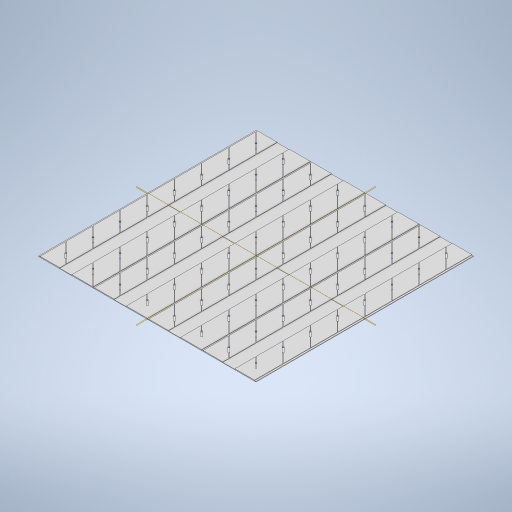
# Autodesk Inventor part: Board ReedSwitchHolder
Saved by Autodesk Inventor 2023 (Build 270158000, 158)
## iProperties
Created: 2023-04-27
Part Number: Board ReedSwitchHolder
Material: Generic
Document SubType Name: Modeling
Designer: ethan
Density: 1 g/cm^3
Appearance: Default
Author: ethan
Autodesk Inventor part; units mm, degrees
ref_plane "YZ Plane" through (0, 0, 0) normal (1, 0, 0) x (0, 1, 0)
ref_plane "XZ Plane" through (0, 0, 0) normal (0, 1, 0) x (-1, 0, 0)
ref_plane "XY Plane" through (0, 0, 0) normal (0, 0, 1) x (1, 0, 0)
sketch "Sketch1" plane through (0, 0, 0) normal (0, 1, 0) x (-1, 0, 0)
  line L0 (0, 0) -> (-649.6, 0) construction
  line L1 (-649.6, 0) -> (-649.6, -649.6) construction
  line L2 (-649.6, -649.6) -> (0, -649.6) construction
  line L3 (0, -649.6) -> (0, 0) construction
  line L4 (-45.4, -604.2) -> (-604.2, -604.2)
  line L5 (-604.2, -604.2) -> (-604.2, -45.4)
  line L6 (-604.2, -45.4) -> (-45.4, -45.4)
  line L7 (-45.4, -45.4) -> (-45.4, -604.2)
  line L8 (-96.2, -553.4) -> (-153.35, -553.4) construction
  line L9 (-153.35, -553.4) -> (-153.35, -496.25) construction
  line L10 (-153.35, -496.25) -> (-96.2, -496.25) construction
  line L11 (-96.2, -496.25) -> (-96.2, -553.4) construction
  line L12 (-96.2, -553.4) -> (-153.35, -496.25) construction
  line L13 (-118.5878, -529.2444) -> (-120.3556, -531.0122)
  line L14 (-120.3556, -531.0122) -> (-130.9622, -520.4056)
  line L15 (-130.9622, -520.4056) -> (-129.1944, -518.6378)
  line L16 (-129.1944, -518.6378) -> (-118.5878, -529.2444)
  line L17 (-118.5878, -529.2444) -> (-130.9622, -520.4056) construction
  line L18 (-120.3556, -531.0122) -> (-129.1944, -518.6378) construction
  line L19 (-177.5056, -531.0122) -> (-188.1122, -520.4056)
  line L20 (-175.7378, -529.2444) -> (-177.5056, -531.0122)
  line L21 (-186.3444, -518.6378) -> (-175.7378, -529.2444)
  line L22 (-188.1122, -520.4056) -> (-186.3444, -518.6378)
  line L23 (-234.6556, -531.0122) -> (-245.2622, -520.4056)
  line L24 (-232.8878, -529.2444) -> (-234.6556, -531.0122)
  line L25 (-243.4944, -518.6378) -> (-232.8878, -529.2444)
  line L26 (-245.2622, -520.4056) -> (-243.4944, -518.6378)
  line L27 (-291.8056, -531.0122) -> (-302.4122, -520.4056)
  line L28 (-290.0378, -529.2444) -> (-291.8056, -531.0122)
  line L29 (-300.6444, -518.6378) -> (-290.0378, -529.2444)
  line L30 (-302.4122, -520.4056) -> (-300.6444, -518.6378)
  line L31 (-348.9556, -531.0122) -> (-359.5622, -520.4056)
  line L32 (-347.1878, -529.2444) -> (-348.9556, -531.0122)
  line L33 (-357.7944, -518.6378) -> (-347.1878, -529.2444)
  line L34 (-359.5622, -520.4056) -> (-357.7944, -518.6378)
  line L35 (-406.1056, -531.0122) -> (-416.7122, -520.4056)
  line L36 (-404.3378, -529.2444) -> (-406.1056, -531.0122)
  line L37 (-414.9444, -518.6378) -> (-404.3378, -529.2444)
  line L38 (-416.7122, -520.4056) -> (-414.9444, -518.6378)
  line L39 (-463.2556, -531.0122) -> (-473.8622, -520.4056)
  line L40 (-461.4878, -529.2444) -> (-463.2556, -531.0122)
  line L41 (-472.0944, -518.6378) -> (-461.4878, -529.2444)
  line L42 (-473.8622, -520.4056) -> (-472.0944, -518.6378)
  line L43 (-520.4056, -531.0122) -> (-531.0122, -520.4056)
  line L44 (-518.6378, -529.2444) -> (-520.4056, -531.0122)
  line L45 (-529.2444, -518.6378) -> (-518.6378, -529.2444)
  line L46 (-531.0122, -520.4056) -> (-529.2444, -518.6378)
  line L47 (-120.3556, -473.8622) -> (-130.9622, -463.2556)
  line L48 (-118.5878, -472.0944) -> (-120.3556, -473.8622)
  line L49 (-129.1944, -461.4878) -> (-118.5878, -472.0944)
  line L50 (-130.9622, -463.2556) -> (-129.1944, -461.4878)
  line L51 (-177.5056, -473.8622) -> (-188.1122, -463.2556)
  line L52 (-175.7378, -472.0944) -> (-177.5056, -473.8622)
  line L53 (-186.3444, -461.4878) -> (-175.7378, -472.0944)
  line L54 (-188.1122, -463.2556) -> (-186.3444, -461.4878)
  line L55 (-234.6556, -473.8622) -> (-245.2622, -463.2556)
  line L56 (-232.8878, -472.0944) -> (-234.6556, -473.8622)
  line L57 (-243.4944, -461.4878) -> (-232.8878, -472.0944)
  line L58 (-245.2622, -463.2556) -> (-243.4944, -461.4878)
  line L59 (-291.8056, -473.8622) -> (-302.4122, -463.2556)
  line L60 (-290.0378, -472.0944) -> (-291.8056, -473.8622)
  line L61 (-300.6444, -461.4878) -> (-290.0378, -472.0944)
  line L62 (-302.4122, -463.2556) -> (-300.6444, -461.4878)
  line L63 (-348.9556, -473.8622) -> (-359.5622, -463.2556)
  line L64 (-347.1878, -472.0944) -> (-348.9556, -473.8622)
  line L65 (-357.7944, -461.4878) -> (-347.1878, -472.0944)
  line L66 (-359.5622, -463.2556) -> (-357.7944, -461.4878)
  line L67 (-406.1056, -473.8622) -> (-416.7122, -463.2556)
  line L68 (-404.3378, -472.0944) -> (-406.1056, -473.8622)
  line L69 (-414.9444, -461.4878) -> (-404.3378, -472.0944)
  line L70 (-416.7122, -463.2556) -> (-414.9444, -461.4878)
  line L71 (-463.2556, -473.8622) -> (-473.8622, -463.2556)
  line L72 (-461.4878, -472.0944) -> (-463.2556, -473.8622)
  line L73 (-472.0944, -461.4878) -> (-461.4878, -472.0944)
  line L74 (-473.8622, -463.2556) -> (-472.0944, -461.4878)
  line L75 (-520.4056, -473.8622) -> (-531.0122, -463.2556)
  line L76 (-518.6378, -472.0944) -> (-520.4056, -473.8622)
  line L77 (-529.2444, -461.4878) -> (-518.6378, -472.0944)
  line L78 (-531.0122, -463.2556) -> (-529.2444, -461.4878)
  line L79 (-120.3556, -416.7122) -> (-130.9622, -406.1056)
  line L80 (-118.5878, -414.9444) -> (-120.3556, -416.7122)
  line L81 (-129.1944, -404.3378) -> (-118.5878, -414.9444)
  line L82 (-130.9622, -406.1056) -> (-129.1944, -404.3378)
  line L83 (-177.5056, -416.7122) -> (-188.1122, -406.1056)
  line L84 (-175.7378, -414.9444) -> (-177.5056, -416.7122)
  line L85 (-186.3444, -404.3378) -> (-175.7378, -414.9444)
  line L86 (-188.1122, -406.1056) -> (-186.3444, -404.3378)
  line L87 (-234.6556, -416.7122) -> (-245.2622, -406.1056)
  line L88 (-232.8878, -414.9444) -> (-234.6556, -416.7122)
  line L89 (-243.4944, -404.3378) -> (-232.8878, -414.9444)
  line L90 (-245.2622, -406.1056) -> (-243.4944, -404.3378)
  line L91 (-291.8056, -416.7122) -> (-302.4122, -406.1056)
  line L92 (-290.0378, -414.9444) -> (-291.8056, -416.7122)
  line L93 (-300.6444, -404.3378) -> (-290.0378, -414.9444)
  line L94 (-302.4122, -406.1056) -> (-300.6444, -404.3378)
  line L95 (-348.9556, -416.7122) -> (-359.5622, -406.1056)
  line L96 (-347.1878, -414.9444) -> (-348.9556, -416.7122)
  line L97 (-357.7944, -404.3378) -> (-347.1878, -414.9444)
  line L98 (-359.5622, -406.1056) -> (-357.7944, -404.3378)
  line L99 (-406.1056, -416.7122) -> (-416.7122, -406.1056)
  line L100 (-404.3378, -414.9444) -> (-406.1056, -416.7122)
  line L101 (-414.9444, -404.3378) -> (-404.3378, -414.9444)
  line L102 (-416.7122, -406.1056) -> (-414.9444, -404.3378)
  line L103 (-463.2556, -416.7122) -> (-473.8622, -406.1056)
  line L104 (-461.4878, -414.9444) -> (-463.2556, -416.7122)
  line L105 (-472.0944, -404.3378) -> (-461.4878, -414.9444)
  line L106 (-473.8622, -406.1056) -> (-472.0944, -404.3378)
  line L107 (-520.4056, -416.7122) -> (-531.0122, -406.1056)
  line L108 (-518.6378, -414.9444) -> (-520.4056, -416.7122)
  line L109 (-529.2444, -404.3378) -> (-518.6378, -414.9444)
  line L110 (-531.0122, -406.1056) -> (-529.2444, -404.3378)
  line L111 (-120.3556, -359.5622) -> (-130.9622, -348.9556)
  line L112 (-118.5878, -357.7944) -> (-120.3556, -359.5622)
  line L113 (-129.1944, -347.1878) -> (-118.5878, -357.7944)
  line L114 (-130.9622, -348.9556) -> (-129.1944, -347.1878)
  line L115 (-177.5056, -359.5622) -> (-188.1122, -348.9556)
  line L116 (-175.7378, -357.7944) -> (-177.5056, -359.5622)
  line L117 (-186.3444, -347.1878) -> (-175.7378, -357.7944)
  line L118 (-188.1122, -348.9556) -> (-186.3444, -347.1878)
  line L119 (-234.6556, -359.5622) -> (-245.2622, -348.9556)
  line L120 (-232.8878, -357.7944) -> (-234.6556, -359.5622)
  line L121 (-243.4944, -347.1878) -> (-232.8878, -357.7944)
  line L122 (-245.2622, -348.9556) -> (-243.4944, -347.1878)
  line L123 (-291.8056, -359.5622) -> (-302.4122, -348.9556)
  line L124 (-290.0378, -357.7944) -> (-291.8056, -359.5622)
  line L125 (-300.6444, -347.1878) -> (-290.0378, -357.7944)
  line L126 (-302.4122, -348.9556) -> (-300.6444, -347.1878)
  line L127 (-348.9556, -359.5622) -> (-359.5622, -348.9556)
  line L128 (-347.1878, -357.7944) -> (-348.9556, -359.5622)
  line L129 (-357.7944, -347.1878) -> (-347.1878, -357.7944)
  line L130 (-359.5622, -348.9556) -> (-357.7944, -347.1878)
  line L131 (-406.1056, -359.5622) -> (-416.7122, -348.9556)
  line L132 (-404.3378, -357.7944) -> (-406.1056, -359.5622)
  line L133 (-414.9444, -347.1878) -> (-404.3378, -357.7944)
  line L134 (-416.7122, -348.9556) -> (-414.9444, -347.1878)
  line L135 (-463.2556, -359.5622) -> (-473.8622, -348.9556)
  line L136 (-461.4878, -357.7944) -> (-463.2556, -359.5622)
  line L137 (-472.0944, -347.1878) -> (-461.4878, -357.7944)
  line L138 (-473.8622, -348.9556) -> (-472.0944, -347.1878)
  line L139 (-520.4056, -359.5622) -> (-531.0122, -348.9556)
  line L140 (-518.6378, -357.7944) -> (-520.4056, -359.5622)
  line L141 (-529.2444, -347.1878) -> (-518.6378, -357.7944)
  line L142 (-531.0122, -348.9556) -> (-529.2444, -347.1878)
  line L143 (-120.3556, -302.4122) -> (-130.9622, -291.8056)
  line L144 (-118.5878, -300.6444) -> (-120.3556, -302.4122)
  line L145 (-129.1944, -290.0378) -> (-118.5878, -300.6444)
  line L146 (-130.9622, -291.8056) -> (-129.1944, -290.0378)
  line L147 (-177.5056, -302.4122) -> (-188.1122, -291.8056)
  line L148 (-175.7378, -300.6444) -> (-177.5056, -302.4122)
  line L149 (-186.3444, -290.0378) -> (-175.7378, -300.6444)
  line L150 (-188.1122, -291.8056) -> (-186.3444, -290.0378)
  line L151 (-234.6556, -302.4122) -> (-245.2622, -291.8056)
  line L152 (-232.8878, -300.6444) -> (-234.6556, -302.4122)
  line L153 (-243.4944, -290.0378) -> (-232.8878, -300.6444)
  line L154 (-245.2622, -291.8056) -> (-243.4944, -290.0378)
  line L155 (-291.8056, -302.4122) -> (-302.4122, -291.8056)
  line L156 (-290.0378, -300.6444) -> (-291.8056, -302.4122)
  line L157 (-300.6444, -290.0378) -> (-290.0378, -300.6444)
  line L158 (-302.4122, -291.8056) -> (-300.6444, -290.0378)
  line L159 (-348.9556, -302.4122) -> (-359.5622, -291.8056)
  line L160 (-347.1878, -300.6444) -> (-348.9556, -302.4122)
  line L161 (-357.7944, -290.0378) -> (-347.1878, -300.6444)
  line L162 (-359.5622, -291.8056) -> (-357.7944, -290.0378)
  line L163 (-406.1056, -302.4122) -> (-416.7122, -291.8056)
  line L164 (-404.3378, -300.6444) -> (-406.1056, -302.4122)
  line L165 (-414.9444, -290.0378) -> (-404.3378, -300.6444)
  line L166 (-416.7122, -291.8056) -> (-414.9444, -290.0378)
  line L167 (-463.2556, -302.4122) -> (-473.8622, -291.8056)
  line L168 (-461.4878, -300.6444) -> (-463.2556, -302.4122)
  line L169 (-472.0944, -290.0378) -> (-461.4878, -300.6444)
  line L170 (-473.8622, -291.8056) -> (-472.0944, -290.0378)
  line L171 (-520.4056, -302.4122) -> (-531.0122, -291.8056)
  line L172 (-518.6378, -300.6444) -> (-520.4056, -302.4122)
  line L173 (-529.2444, -290.0378) -> (-518.6378, -300.6444)
  line L174 (-531.0122, -291.8056) -> (-529.2444, -290.0378)
  line L175 (-120.3556, -245.2622) -> (-130.9622, -234.6556)
  line L176 (-118.5878, -243.4944) -> (-120.3556, -245.2622)
  line L177 (-129.1944, -232.8878) -> (-118.5878, -243.4944)
  line L178 (-130.9622, -234.6556) -> (-129.1944, -232.8878)
  line L179 (-177.5056, -245.2622) -> (-188.1122, -234.6556)
  line L180 (-175.7378, -243.4944) -> (-177.5056, -245.2622)
  line L181 (-186.3444, -232.8878) -> (-175.7378, -243.4944)
  line L182 (-188.1122, -234.6556) -> (-186.3444, -232.8878)
  line L183 (-234.6556, -245.2622) -> (-245.2622, -234.6556)
  line L184 (-232.8878, -243.4944) -> (-234.6556, -245.2622)
  line L185 (-243.4944, -232.8878) -> (-232.8878, -243.4944)
  line L186 (-245.2622, -234.6556) -> (-243.4944, -232.8878)
  line L187 (-291.8056, -245.2622) -> (-302.4122, -234.6556)
  line L188 (-290.0378, -243.4944) -> (-291.8056, -245.2622)
  line L189 (-300.6444, -232.8878) -> (-290.0378, -243.4944)
  line L190 (-302.4122, -234.6556) -> (-300.6444, -232.8878)
  line L191 (-348.9556, -245.2622) -> (-359.5622, -234.6556)
  line L192 (-347.1878, -243.4944) -> (-348.9556, -245.2622)
  line L193 (-357.7944, -232.8878) -> (-347.1878, -243.4944)
  line L194 (-359.5622, -234.6556) -> (-357.7944, -232.8878)
  line L195 (-406.1056, -245.2622) -> (-416.7122, -234.6556)
  line L196 (-404.3378, -243.4944) -> (-406.1056, -245.2622)
  line L197 (-414.9444, -232.8878) -> (-404.3378, -243.4944)
  line L198 (-416.7122, -234.6556) -> (-414.9444, -232.8878)
  line L199 (-463.2556, -245.2622) -> (-473.8622, -234.6556)
  line L200 (-461.4878, -243.4944) -> (-463.2556, -245.2622)
  line L201 (-472.0944, -232.8878) -> (-461.4878, -243.4944)
  line L202 (-473.8622, -234.6556) -> (-472.0944, -232.8878)
  line L203 (-520.4056, -245.2622) -> (-531.0122, -234.6556)
  line L204 (-518.6378, -243.4944) -> (-520.4056, -245.2622)
  line L205 (-529.2444, -232.8878) -> (-518.6378, -243.4944)
  line L206 (-531.0122, -234.6556) -> (-529.2444, -232.8878)
  line L207 (-120.3556, -188.1122) -> (-130.9622, -177.5056)
  line L208 (-118.5878, -186.3444) -> (-120.3556, -188.1122)
  line L209 (-129.1944, -175.7378) -> (-118.5878, -186.3444)
  line L210 (-130.9622, -177.5056) -> (-129.1944, -175.7378)
  line L211 (-177.5056, -188.1122) -> (-188.1122, -177.5056)
  line L212 (-175.7378, -186.3444) -> (-177.5056, -188.1122)
  line L213 (-186.3444, -175.7378) -> (-175.7378, -186.3444)
  line L214 (-188.1122, -177.5056) -> (-186.3444, -175.7378)
  line L215 (-234.6556, -188.1122) -> (-245.2622, -177.5056)
  line L216 (-232.8878, -186.3444) -> (-234.6556, -188.1122)
  line L217 (-243.4944, -175.7378) -> (-232.8878, -186.3444)
  line L218 (-245.2622, -177.5056) -> (-243.4944, -175.7378)
  line L219 (-291.8056, -188.1122) -> (-302.4122, -177.5056)
  line L220 (-290.0378, -186.3444) -> (-291.8056, -188.1122)
  line L221 (-300.6444, -175.7378) -> (-290.0378, -186.3444)
  line L222 (-302.4122, -177.5056) -> (-300.6444, -175.7378)
  line L223 (-348.9556, -188.1122) -> (-359.5622, -177.5056)
  line L224 (-347.1878, -186.3444) -> (-348.9556, -188.1122)
  line L225 (-357.7944, -175.7378) -> (-347.1878, -186.3444)
  line L226 (-359.5622, -177.5056) -> (-357.7944, -175.7378)
  line L227 (-406.1056, -188.1122) -> (-416.7122, -177.5056)
  line L228 (-404.3378, -186.3444) -> (-406.1056, -188.1122)
  line L229 (-414.9444, -175.7378) -> (-404.3378, -186.3444)
  line L230 (-416.7122, -177.5056) -> (-414.9444, -175.7378)
  line L231 (-463.2556, -188.1122) -> (-473.8622, -177.5056)
  line L232 (-461.4878, -186.3444) -> (-463.2556, -188.1122)
  line L233 (-472.0944, -175.7378) -> (-461.4878, -186.3444)
  line L234 (-473.8622, -177.5056) -> (-472.0944, -175.7378)
  line L235 (-520.4056, -188.1122) -> (-531.0122, -177.5056)
  line L236 (-518.6378, -186.3444) -> (-520.4056, -188.1122)
  line L237 (-529.2444, -175.7378) -> (-518.6378, -186.3444)
  line L238 (-531.0122, -177.5056) -> (-529.2444, -175.7378)
  line L239 (-120.3556, -130.9622) -> (-130.9622, -120.3556)
  line L240 (-118.5878, -129.1944) -> (-120.3556, -130.9622)
  line L241 (-129.1944, -118.5878) -> (-118.5878, -129.1944)
  line L242 (-130.9622, -120.3556) -> (-129.1944, -118.5878)
  line L243 (-177.5056, -130.9622) -> (-188.1122, -120.3556)
  line L244 (-175.7378, -129.1944) -> (-177.5056, -130.9622)
  line L245 (-186.3444, -118.5878) -> (-175.7378, -129.1944)
  line L246 (-188.1122, -120.3556) -> (-186.3444, -118.5878)
  line L247 (-234.6556, -130.9622) -> (-245.2622, -120.3556)
  line L248 (-232.8878, -129.1944) -> (-234.6556, -130.9622)
  line L249 (-243.4944, -118.5878) -> (-232.8878, -129.1944)
  line L250 (-245.2622, -120.3556) -> (-243.4944, -118.5878)
  line L251 (-291.8056, -130.9622) -> (-302.4122, -120.3556)
  line L252 (-290.0378, -129.1944) -> (-291.8056, -130.9622)
  line L253 (-300.6444, -118.5878) -> (-290.0378, -129.1944)
  line L254 (-302.4122, -120.3556) -> (-300.6444, -118.5878)
  line L255 (-348.9556, -130.9622) -> (-359.5622, -120.3556)
  line L256 (-347.1878, -129.1944) -> (-348.9556, -130.9622)
  line L257 (-357.7944, -118.5878) -> (-347.1878, -129.1944)
  line L258 (-359.5622, -120.3556) -> (-357.7944, -118.5878)
  line L259 (-406.1056, -130.9622) -> (-416.7122, -120.3556)
  line L260 (-404.3378, -129.1944) -> (-406.1056, -130.9622)
  line L261 (-414.9444, -118.5878) -> (-404.3378, -129.1944)
  line L262 (-416.7122, -120.3556) -> (-414.9444, -118.5878)
  line L263 (-463.2556, -130.9622) -> (-473.8622, -120.3556)
  line L264 (-461.4878, -129.1944) -> (-463.2556, -130.9622)
  line L265 (-472.0944, -118.5878) -> (-461.4878, -129.1944)
  line L266 (-473.8622, -120.3556) -> (-472.0944, -118.5878)
  line L267 (-520.4056, -130.9622) -> (-531.0122, -120.3556)
  line L268 (-518.6378, -129.1944) -> (-520.4056, -130.9622)
  line L269 (-529.2444, -118.5878) -> (-518.6378, -129.1944)
  line L270 (-531.0122, -120.3556) -> (-529.2444, -118.5878)
  line L271 (-96.2, -553.4) -> (-553.4, -553.4)
  line L272 (-553.4, -553.4) -> (-553.4, -96.2)
  line L273 (-553.4, -96.2) -> (-96.2, -96.2)
  line L274 (-96.2, -96.2) -> (-96.2, -553.4)
  line L275 (-553.4, -324.8) -> (-96.2, -324.8)
  line L276 (-324.8, -553.4) -> (-324.8, -96.2)
  point P0 (-124.775, -524.825)
  dimension "d0" = 649.6
  dimension "d1" = 649.6
  dimension "d10" = 45.4
  dimension "d11" = 50.8
  dimension "d12" = 50.8
  dimension "d15" = 57.15
  dimension "d16" = 57.15
  dimension "d17" = 2.5
  dimension "d18" = 15
  dimension "d22" = 57.15
  dimension "d25" = 57.15
  dimension "d30" = 50.8
  constraints: 554 end point, 10 parallel, 7 midpoint, 6 perpendicular, 3 horizontal, 1 vertical, 510 other
  measures "d0" distance of L2.end L1.end
  measures "d1" distance of L1.end L0.end
  measures "d10" distance between parallel lines of L2 L4
  measures "d11" distance from line of L4 L8.start
  measures "d12" distance from line of L7 L8.start
  measures "d15" distance of L9.end L10.end
  measures "d16" distance of L8.end L9.end
  measures "d17" distance of L13.start L13.end
  measures "d18" distance of L13.end L14.end
  measures "d22" distance of L13.end L19.start
  measures "d25" distance of L13.end L47.start
  measures "d30" distance between parallel lines of L7 L274
extrude "Extrusion1" add sketch "Sketch1" along normal blind 2 contours L271 L276 L275 L274 | L271 L272 L275 L276 | L275 L276 L273 L274 | L275 L272 L273 L276
sketch "Sketch2" plane through (0, 2, 0) normal (0, 1, 0) x (1, 0, 0)
  line L0 (553.4, 553.4) -> (96.2, 553.4) projected
  line L1 (96.2, 553.4) -> (99.375, 553.4)
  line L2 (99.375, 553.4) -> (99.375, 96.2)
  line L3 (99.375, 96.2) -> (96.2, 96.2)
  line L4 (96.2, 96.2) -> (96.2, 553.4)
  line L5 (553.4, 96.2) -> (553.4, 553.4) projected
  line L6 (140.65, 553.4) -> (166.05, 553.4)
  line L7 (166.05, 553.4) -> (166.05, 96.2)
  line L8 (166.05, 96.2) -> (140.65, 96.2)
  line L9 (140.65, 96.2) -> (140.65, 553.4)
  line L10 (280.35, 553.4) -> (280.35, 96.2)
  line L11 (254.95, 96.2) -> (254.95, 553.4)
  line L12 (254.95, 553.4) -> (280.35, 553.4)
  line L13 (213.675, 553.4) -> (213.675, 96.2)
  line L14 (210.5, 96.2) -> (210.5, 553.4)
  line L15 (210.5, 553.4) -> (213.675, 553.4)
  line L16 (280.35, 96.2) -> (254.95, 96.2)
  line L17 (213.675, 96.2) -> (210.5, 96.2)
  line L18 (394.65, 553.4) -> (394.65, 96.2)
  line L19 (369.25, 96.2) -> (369.25, 553.4)
  line L20 (369.25, 553.4) -> (394.65, 553.4)
  line L21 (327.975, 553.4) -> (327.975, 96.2)
  line L22 (324.8, 96.2) -> (324.8, 553.4)
  line L23 (324.8, 553.4) -> (327.975, 553.4)
  line L24 (394.65, 96.2) -> (369.25, 96.2)
  line L25 (327.975, 96.2) -> (324.8, 96.2)
  line L26 (508.95, 553.4) -> (508.95, 96.2)
  line L27 (483.55, 96.2) -> (483.55, 553.4)
  line L28 (483.55, 553.4) -> (508.95, 553.4)
  line L29 (442.275, 553.4) -> (442.275, 96.2)
  line L30 (439.1, 96.2) -> (439.1, 553.4)
  line L31 (439.1, 553.4) -> (442.275, 553.4)
  line L32 (508.95, 96.2) -> (483.55, 96.2)
  line L33 (442.275, 96.2) -> (439.1, 96.2)
  line L34 (553.4, 553.4) -> (550.225, 553.4)
  line L35 (550.225, 553.4) -> (550.225, 96.2)
  line L36 (550.225, 96.2) -> (553.4, 96.2)
  line L37 (553.4, 96.2) -> (553.4, 553.4)
  line L38 (118.5878, 529.2444) -> (120.3556, 531.0122) construction
  line L39 (119.4717, 530.1283) -> (99.375, 550.225) construction
  line L40 (130.9622, 520.4056) -> (129.1944, 518.6378) construction
  line L41 (130.0783, 519.5217) -> (140.65, 508.95) construction
  line L42 (119.8253, 530.4819) -> (99.375, 550.9321)
  line L43 (119.1181, 529.7747) -> (99.375, 549.5179)
  line L44 (130.4319, 519.8753) -> (140.65, 509.6571)
  line L45 (129.7247, 519.1681) -> (140.65, 508.2429)
  line L46 (118.5878, 529.2444) -> (120.3556, 531.0122) construction
  line L47 (130.9622, 520.4056) -> (129.1944, 518.6378) construction
  line L48 (234.1253, 530.4819) -> (213.675, 550.9321)
  line L49 (233.4181, 529.7747) -> (213.675, 549.5179)
  line L50 (244.7319, 519.8753) -> (254.95, 509.6571)
  line L51 (244.0247, 519.1681) -> (254.95, 508.2429)
  line L52 (348.4253, 530.4819) -> (327.975, 550.9321)
  line L53 (347.7181, 529.7747) -> (327.975, 549.5179)
  line L54 (359.0319, 519.8753) -> (369.25, 509.6571)
  line L55 (358.3247, 519.1681) -> (369.25, 508.2429)
  line L56 (462.7253, 530.4819) -> (442.275, 550.9321)
  line L57 (462.0181, 529.7747) -> (442.275, 549.5179)
  line L58 (473.3319, 519.8753) -> (483.55, 509.6571)
  line L59 (472.6247, 519.1681) -> (483.55, 508.2429)
  line L60 (119.8253, 473.3319) -> (99.375, 493.7821)
  line L61 (119.1181, 472.6247) -> (99.375, 492.3679)
  line L62 (130.4319, 462.7253) -> (140.65, 452.5071)
  line L63 (129.7247, 462.0181) -> (140.65, 451.0929)
  line L64 (234.1253, 473.3319) -> (213.675, 493.7821)
  line L65 (233.4181, 472.6247) -> (213.675, 492.3679)
  line L66 (244.7319, 462.7253) -> (254.95, 452.5071)
  line L67 (244.0247, 462.0181) -> (254.95, 451.0929)
  line L68 (348.4253, 473.3319) -> (327.975, 493.7821)
  line L69 (347.7181, 472.6247) -> (327.975, 492.3679)
  line L70 (359.0319, 462.7253) -> (369.25, 452.5071)
  line L71 (358.3247, 462.0181) -> (369.25, 451.0929)
  line L72 (462.7253, 473.3319) -> (442.275, 493.7821)
  line L73 (462.0181, 472.6247) -> (442.275, 492.3679)
  line L74 (473.3319, 462.7253) -> (483.55, 452.5071)
  line L75 (472.6247, 462.0181) -> (483.55, 451.0929)
  line L76 (119.8253, 416.1819) -> (99.375, 436.6321)
  line L77 (119.1181, 415.4747) -> (99.375, 435.2179)
  line L78 (130.4319, 405.5753) -> (140.65, 395.3571)
  line L79 (129.7247, 404.8681) -> (140.65, 393.9429)
  line L80 (234.1253, 416.1819) -> (213.675, 436.6321)
  line L81 (233.4181, 415.4747) -> (213.675, 435.2179)
  line L82 (244.7319, 405.5753) -> (254.95, 395.3571)
  line L83 (244.0247, 404.8681) -> (254.95, 393.9429)
  line L84 (348.4253, 416.1819) -> (327.975, 436.6321)
  line L85 (347.7181, 415.4747) -> (327.975, 435.2179)
  line L86 (359.0319, 405.5753) -> (369.25, 395.3571)
  line L87 (358.3247, 404.8681) -> (369.25, 393.9429)
  line L88 (462.7253, 416.1819) -> (442.275, 436.6321)
  line L89 (462.0181, 415.4747) -> (442.275, 435.2179)
  line L90 (473.3319, 405.5753) -> (483.55, 395.3571)
  line L91 (472.6247, 404.8681) -> (483.55, 393.9429)
  line L92 (119.8253, 359.0319) -> (99.375, 379.4821)
  line L93 (119.1181, 358.3247) -> (99.375, 378.0679)
  line L94 (130.4319, 348.4253) -> (140.65, 338.2071)
  line L95 (129.7247, 347.7181) -> (140.65, 336.7929)
  line L96 (234.1253, 359.0319) -> (213.675, 379.4821)
  line L97 (233.4181, 358.3247) -> (213.675, 378.0679)
  line L98 (244.7319, 348.4253) -> (254.95, 338.2071)
  line L99 (244.0247, 347.7181) -> (254.95, 336.7929)
  line L100 (348.4253, 359.0319) -> (327.975, 379.4821)
  line L101 (347.7181, 358.3247) -> (327.975, 378.0679)
  line L102 (359.0319, 348.4253) -> (369.25, 338.2071)
  line L103 (358.3247, 347.7181) -> (369.25, 336.7929)
  line L104 (462.7253, 359.0319) -> (442.275, 379.4821)
  line L105 (462.0181, 358.3247) -> (442.275, 378.0679)
  line L106 (473.3319, 348.4253) -> (483.55, 338.2071)
  line L107 (472.6247, 347.7181) -> (483.55, 336.7929)
  line L108 (119.8253, 301.8819) -> (99.375, 322.3321)
  line L109 (119.1181, 301.1747) -> (99.375, 320.9179)
  line L110 (130.4319, 291.2753) -> (140.65, 281.0571)
  line L111 (129.7247, 290.5681) -> (140.65, 279.6429)
  line L112 (234.1253, 301.8819) -> (213.675, 322.3321)
  line L113 (233.4181, 301.1747) -> (213.675, 320.9179)
  line L114 (244.7319, 291.2753) -> (254.95, 281.0571)
  line L115 (244.0247, 290.5681) -> (254.95, 279.6429)
  line L116 (348.4253, 301.8819) -> (327.975, 322.3321)
  line L117 (347.7181, 301.1747) -> (327.975, 320.9179)
  line L118 (359.0319, 291.2753) -> (369.25, 281.0571)
  line L119 (358.3247, 290.5681) -> (369.25, 279.6429)
  line L120 (462.7253, 301.8819) -> (442.275, 322.3321)
  line L121 (462.0181, 301.1747) -> (442.275, 320.9179)
  line L122 (473.3319, 291.2753) -> (483.55, 281.0571)
  line L123 (472.6247, 290.5681) -> (483.55, 279.6429)
  line L124 (119.8253, 244.7319) -> (99.375, 265.1821)
  line L125 (119.1181, 244.0247) -> (99.375, 263.7679)
  line L126 (130.4319, 234.1253) -> (140.65, 223.9071)
  line L127 (129.7247, 233.4181) -> (140.65, 222.4929)
  line L128 (234.1253, 244.7319) -> (213.675, 265.1821)
  line L129 (233.4181, 244.0247) -> (213.675, 263.7679)
  line L130 (244.7319, 234.1253) -> (254.95, 223.9071)
  line L131 (244.0247, 233.4181) -> (254.95, 222.4929)
  line L132 (348.4253, 244.7319) -> (327.975, 265.1821)
  line L133 (347.7181, 244.0247) -> (327.975, 263.7679)
  line L134 (359.0319, 234.1253) -> (369.25, 223.9071)
  line L135 (358.3247, 233.4181) -> (369.25, 222.4929)
  line L136 (462.7253, 244.7319) -> (442.275, 265.1821)
  line L137 (462.0181, 244.0247) -> (442.275, 263.7679)
  line L138 (473.3319, 234.1253) -> (483.55, 223.9071)
  line L139 (472.6247, 233.4181) -> (483.55, 222.4929)
  line L140 (119.8253, 187.5819) -> (99.375, 208.0321)
  line L141 (119.1181, 186.8747) -> (99.375, 206.6179)
  line L142 (130.4319, 176.9753) -> (140.65, 166.7571)
  line L143 (129.7247, 176.2681) -> (140.65, 165.3429)
  line L144 (234.1253, 187.5819) -> (213.675, 208.0321)
  line L145 (233.4181, 186.8747) -> (213.675, 206.6179)
  line L146 (244.7319, 176.9753) -> (254.95, 166.7571)
  line L147 (244.0247, 176.2681) -> (254.95, 165.3429)
  line L148 (348.4253, 187.5819) -> (327.975, 208.0321)
  line L149 (347.7181, 186.8747) -> (327.975, 206.6179)
  line L150 (359.0319, 176.9753) -> (369.25, 166.7571)
  line L151 (358.3247, 176.2681) -> (369.25, 165.3429)
  line L152 (462.7253, 187.5819) -> (442.275, 208.0321)
  line L153 (462.0181, 186.8747) -> (442.275, 206.6179)
  line L154 (473.3319, 176.9753) -> (483.55, 166.7571)
  line L155 (472.6247, 176.2681) -> (483.55, 165.3429)
  line L156 (119.8253, 130.4319) -> (99.375, 150.8821)
  line L157 (119.1181, 129.7247) -> (99.375, 149.4679)
  line L158 (130.4319, 119.8253) -> (140.65, 109.6071)
  line L159 (129.7247, 119.1181) -> (140.65, 108.1929)
  line L160 (234.1253, 130.4319) -> (213.675, 150.8821)
  line L161 (233.4181, 129.7247) -> (213.675, 149.4679)
  line L162 (244.7319, 119.8253) -> (254.95, 109.6071)
  line L163 (244.0247, 119.1181) -> (254.95, 108.1929)
  line L164 (348.4253, 130.4319) -> (327.975, 150.8821)
  line L165 (347.7181, 129.7247) -> (327.975, 149.4679)
  line L166 (359.0319, 119.8253) -> (369.25, 109.6071)
  line L167 (358.3247, 119.1181) -> (369.25, 108.1929)
  line L168 (462.7253, 130.4319) -> (442.275, 150.8821)
  line L169 (462.0181, 129.7247) -> (442.275, 149.4679)
  line L170 (473.3319, 119.8253) -> (483.55, 109.6071)
  line L171 (472.6247, 119.1181) -> (483.55, 108.1929)
  line L172 (175.7378, 529.2444) -> (177.5056, 531.0122) construction
  line L173 (176.6217, 530.1283) -> (166.05, 540.7) construction
  line L174 (188.1122, 520.4056) -> (186.3444, 518.6378) construction
  line L175 (187.2283, 519.5217) -> (210.5, 496.25) construction
  line L176 (176.9753, 530.4819) -> (166.05, 541.4071)
  line L177 (176.2681, 529.7747) -> (166.05, 539.9929)
  line L178 (187.5819, 519.8753) -> (210.5, 496.9571)
  line L179 (186.8747, 519.1681) -> (210.5, 495.5429)
  line L180 (291.2753, 530.4819) -> (280.35, 541.4071)
  line L181 (290.5681, 529.7747) -> (280.35, 539.9929)
  line L182 (301.8819, 519.8753) -> (324.8, 496.9571)
  line L183 (301.1747, 519.1681) -> (324.8, 495.5429)
  line L184 (405.5753, 530.4819) -> (394.65, 541.4071)
  line L185 (404.8681, 529.7747) -> (394.65, 539.9929)
  line L186 (416.1819, 519.8753) -> (439.1, 496.9571)
  line L187 (415.4747, 519.1681) -> (439.1, 495.5429)
  line L188 (519.8753, 530.4819) -> (508.95, 541.4071)
  line L189 (519.1681, 529.7747) -> (508.95, 539.9929)
  line L190 (530.4819, 519.8753) -> (553.4, 496.9571)
  line L191 (529.7747, 519.1681) -> (553.4, 495.5429)
  line L192 (176.9753, 473.3319) -> (166.05, 484.2571)
  line L193 (176.2681, 472.6247) -> (166.05, 482.8429)
  line L194 (187.5819, 462.7253) -> (210.5, 439.8071)
  line L195 (186.8747, 462.0181) -> (210.5, 438.3929)
  line L196 (291.2753, 473.3319) -> (280.35, 484.2571)
  line L197 (290.5681, 472.6247) -> (280.35, 482.8429)
  line L198 (301.8819, 462.7253) -> (324.8, 439.8071)
  line L199 (301.1747, 462.0181) -> (324.8, 438.3929)
  line L200 (405.5753, 473.3319) -> (394.65, 484.2571)
  line L201 (404.8681, 472.6247) -> (394.65, 482.8429)
  line L202 (416.1819, 462.7253) -> (439.1, 439.8071)
  line L203 (415.4747, 462.0181) -> (439.1, 438.3929)
  line L204 (519.8753, 473.3319) -> (508.95, 484.2571)
  line L205 (519.1681, 472.6247) -> (508.95, 482.8429)
  line L206 (530.4819, 462.7253) -> (553.4, 439.8071)
  line L207 (529.7747, 462.0181) -> (553.4, 438.3929)
  line L208 (176.9753, 416.1819) -> (166.05, 427.1071)
  line L209 (176.2681, 415.4747) -> (166.05, 425.6929)
  line L210 (187.5819, 405.5753) -> (210.5, 382.6571)
  line L211 (186.8747, 404.8681) -> (210.5, 381.2429)
  line L212 (291.2753, 416.1819) -> (280.35, 427.1071)
  line L213 (290.5681, 415.4747) -> (280.35, 425.6929)
  line L214 (301.8819, 405.5753) -> (324.8, 382.6571)
  line L215 (301.1747, 404.8681) -> (324.8, 381.2429)
  line L216 (405.5753, 416.1819) -> (394.65, 427.1071)
  line L217 (404.8681, 415.4747) -> (394.65, 425.6929)
  line L218 (416.1819, 405.5753) -> (439.1, 382.6571)
  line L219 (415.4747, 404.8681) -> (439.1, 381.2429)
  line L220 (519.8753, 416.1819) -> (508.95, 427.1071)
  line L221 (519.1681, 415.4747) -> (508.95, 425.6929)
  line L222 (530.4819, 405.5753) -> (553.4, 382.6571)
  line L223 (529.7747, 404.8681) -> (553.4, 381.2429)
  line L224 (176.9753, 359.0319) -> (166.05, 369.9571)
  line L225 (176.2681, 358.3247) -> (166.05, 368.5429)
  line L226 (187.5819, 348.4253) -> (210.5, 325.5071)
  line L227 (186.8747, 347.7181) -> (210.5, 324.0929)
  line L228 (291.2753, 359.0319) -> (280.35, 369.9571)
  line L229 (290.5681, 358.3247) -> (280.35, 368.5429)
  line L230 (301.8819, 348.4253) -> (324.8, 325.5071)
  line L231 (301.1747, 347.7181) -> (324.8, 324.0929)
  line L232 (405.5753, 359.0319) -> (394.65, 369.9571)
  line L233 (404.8681, 358.3247) -> (394.65, 368.5429)
  line L234 (416.1819, 348.4253) -> (439.1, 325.5071)
  line L235 (415.4747, 347.7181) -> (439.1, 324.0929)
  line L236 (519.8753, 359.0319) -> (508.95, 369.9571)
  line L237 (519.1681, 358.3247) -> (508.95, 368.5429)
  line L238 (530.4819, 348.4253) -> (553.4, 325.5071)
  line L239 (529.7747, 347.7181) -> (553.4, 324.0929)
  line L240 (176.9753, 301.8819) -> (166.05, 312.8071)
  line L241 (176.2681, 301.1747) -> (166.05, 311.3929)
  line L242 (187.5819, 291.2753) -> (210.5, 268.3571)
  line L243 (186.8747, 290.5681) -> (210.5, 266.9429)
  line L244 (291.2753, 301.8819) -> (280.35, 312.8071)
  line L245 (290.5681, 301.1747) -> (280.35, 311.3929)
  line L246 (301.8819, 291.2753) -> (324.8, 268.3571)
  line L247 (301.1747, 290.5681) -> (324.8, 266.9429)
  line L248 (405.5753, 301.8819) -> (394.65, 312.8071)
  line L249 (404.8681, 301.1747) -> (394.65, 311.3929)
  line L250 (416.1819, 291.2753) -> (439.1, 268.3571)
  line L251 (415.4747, 290.5681) -> (439.1, 266.9429)
  line L252 (519.8753, 301.8819) -> (508.95, 312.8071)
  line L253 (519.1681, 301.1747) -> (508.95, 311.3929)
  line L254 (530.4819, 291.2753) -> (553.4, 268.3571)
  line L255 (529.7747, 290.5681) -> (553.4, 266.9429)
  line L256 (176.9753, 244.7319) -> (166.05, 255.6571)
  line L257 (176.2681, 244.0247) -> (166.05, 254.2429)
  line L258 (187.5819, 234.1253) -> (210.5, 211.2071)
  line L259 (186.8747, 233.4181) -> (210.5, 209.7929)
  line L260 (291.2753, 244.7319) -> (280.35, 255.6571)
  line L261 (290.5681, 244.0247) -> (280.35, 254.2429)
  line L262 (301.8819, 234.1253) -> (324.8, 211.2071)
  line L263 (301.1747, 233.4181) -> (324.8, 209.7929)
  line L264 (405.5753, 244.7319) -> (394.65, 255.6571)
  line L265 (404.8681, 244.0247) -> (394.65, 254.2429)
  line L266 (416.1819, 234.1253) -> (439.1, 211.2071)
  line L267 (415.4747, 233.4181) -> (439.1, 209.7929)
  line L268 (519.8753, 244.7319) -> (508.95, 255.6571)
  line L269 (519.1681, 244.0247) -> (508.95, 254.2429)
  line L270 (530.4819, 234.1253) -> (553.4, 211.2071)
  line L271 (529.7747, 233.4181) -> (553.4, 209.7929)
  line L272 (176.9753, 187.5819) -> (166.05, 198.5071)
  line L273 (176.2681, 186.8747) -> (166.05, 197.0929)
  line L274 (187.5819, 176.9753) -> (210.5, 154.0571)
  line L275 (186.8747, 176.2681) -> (210.5, 152.6429)
  line L276 (291.2753, 187.5819) -> (280.35, 198.5071)
  line L277 (290.5681, 186.8747) -> (280.35, 197.0929)
  line L278 (301.8819, 176.9753) -> (324.8, 154.0571)
  line L279 (301.1747, 176.2681) -> (324.8, 152.6429)
  line L280 (405.5753, 187.5819) -> (394.65, 198.5071)
  line L281 (404.8681, 186.8747) -> (394.65, 197.0929)
  line L282 (416.1819, 176.9753) -> (439.1, 154.0571)
  line L283 (415.4747, 176.2681) -> (439.1, 152.6429)
  line L284 (519.8753, 187.5819) -> (508.95, 198.5071)
  line L285 (519.1681, 186.8747) -> (508.95, 197.0929)
  line L286 (530.4819, 176.9753) -> (553.4, 154.0571)
  line L287 (529.7747, 176.2681) -> (553.4, 152.6429)
  line L288 (176.9753, 130.4319) -> (166.05, 141.3571)
  line L289 (176.2681, 129.7247) -> (166.05, 139.9429)
  line L290 (187.5819, 119.8253) -> (210.5, 96.9071)
  line L291 (186.8747, 119.1181) -> (210.5, 95.4929)
  line L292 (291.2753, 130.4319) -> (280.35, 141.3571)
  line L293 (290.5681, 129.7247) -> (280.35, 139.9429)
  line L294 (301.8819, 119.8253) -> (324.8, 96.9071)
  line L295 (301.1747, 119.1181) -> (324.8, 95.4929)
  line L296 (405.5753, 130.4319) -> (394.65, 141.3571)
  line L297 (404.8681, 129.7247) -> (394.65, 139.9429)
  line L298 (416.1819, 119.8253) -> (439.1, 96.9071)
  line L299 (415.4747, 119.1181) -> (439.1, 95.4929)
  line L300 (519.8753, 130.4319) -> (508.95, 141.3571)
  line L301 (519.1681, 129.7247) -> (508.95, 139.9429)
  line L302 (530.4819, 119.8253) -> (553.4, 96.9071)
  line L303 (529.7747, 119.1181) -> (553.4, 95.4929)
  line L304 (119.1181, 529.7747) -> (119.8253, 530.4819)
  line L305 (129.7247, 519.1681) -> (130.4319, 519.8753)
  line L306 (119.1181, 472.6247) -> (119.8253, 473.3319)
  line L307 (118.5878, 472.0944) -> (120.3556, 473.8622) projected
  line L308 (129.7247, 462.0181) -> (130.4319, 462.7253)
  line L309 (130.9622, 463.2556) -> (129.1944, 461.4878) projected
  line L310 (119.1181, 415.4747) -> (119.8253, 416.1819)
  line L311 (118.5878, 414.9444) -> (120.3556, 416.7122) projected
  line L312 (129.7247, 404.8681) -> (130.4319, 405.5753)
  line L313 (130.9622, 406.1056) -> (129.1944, 404.3378) projected
  line L314 (119.1181, 358.3247) -> (119.8253, 359.0319)
  line L315 (118.5878, 357.7944) -> (120.3556, 359.5622) projected
  line L316 (129.7247, 347.7181) -> (130.4319, 348.4253)
  line L317 (129.1944, 347.1878) -> (118.5878, 357.7944) projected
  line L318 (119.1181, 301.1747) -> (119.8253, 301.8819)
  line L319 (118.5878, 300.6444) -> (120.3556, 302.4122) projected
  line L320 (129.7247, 290.5681) -> (130.4319, 291.2753)
  line L321 (130.9622, 291.8056) -> (129.1944, 290.0378) projected
  line L322 (119.1181, 244.0247) -> (119.8253, 244.7319)
  line L323 (118.5878, 243.4944) -> (120.3556, 245.2622) projected
  line L324 (129.7247, 233.4181) -> (130.4319, 234.1253)
  line L325 (130.9622, 234.6556) -> (129.1944, 232.8878) projected
  line L326 (119.1181, 186.8747) -> (119.8253, 187.5819)
  line L327 (129.1944, 175.7378) -> (118.5878, 186.3444) projected
  line L328 (129.7247, 176.2681) -> (130.4319, 176.9753)
  line L329 (130.9622, 177.5056) -> (129.1944, 175.7378) projected
  line L330 (119.1181, 129.7247) -> (119.8253, 130.4319)
  line L331 (118.5878, 129.1944) -> (120.3556, 130.9622) projected
  line L332 (129.7247, 119.1181) -> (130.4319, 119.8253)
  line L333 (130.9622, 120.3556) -> (129.1944, 118.5878) projected
  line L334 (176.2681, 529.7747) -> (176.9753, 530.4819)
  line L335 (175.7378, 529.2444) -> (177.5056, 531.0122) projected
  line L336 (186.8747, 519.1681) -> (187.5819, 519.8753)
  line L337 (188.1122, 520.4056) -> (186.3444, 518.6378) projected
  line L338 (176.2681, 472.6247) -> (176.9753, 473.3319)
  line L339 (175.7378, 472.0944) -> (177.5056, 473.8622) projected
  line L340 (186.8747, 462.0181) -> (187.5819, 462.7253)
  line L341 (188.1122, 463.2556) -> (186.3444, 461.4878) projected
  line L342 (176.2681, 415.4747) -> (176.9753, 416.1819)
  line L343 (175.7378, 414.9444) -> (177.5056, 416.7122) projected
  line L344 (186.8747, 404.8681) -> (187.5819, 405.5753)
  line L345 (188.1122, 406.1056) -> (186.3444, 404.3378) projected
  line L346 (176.2681, 358.3247) -> (176.9753, 359.0319)
  line L347 (186.8747, 347.7181) -> (187.5819, 348.4253)
  line L348 (188.1122, 348.9556) -> (186.3444, 347.1878) projected
  line L349 (176.2681, 301.1747) -> (176.9753, 301.8819)
  line L350 (175.7378, 300.6444) -> (177.5056, 302.4122) projected
  line L351 (186.8747, 290.5681) -> (187.5819, 291.2753)
  line L352 (188.1122, 291.8056) -> (186.3444, 290.0378) projected
  line L353 (176.2681, 244.0247) -> (176.9753, 244.7319)
  line L354 (175.7378, 243.4944) -> (177.5056, 245.2622) projected
  line L355 (186.8747, 233.4181) -> (187.5819, 234.1253)
  line L356 (188.1122, 234.6556) -> (186.3444, 232.8878) projected
  line L357 (176.2681, 186.8747) -> (176.9753, 187.5819)
  line L358 (175.7378, 186.3444) -> (177.5056, 188.1122) projected
  line L359 (188.1122, 177.5056) -> (186.3444, 175.7378) projected
  line L360 (176.2681, 129.7247) -> (176.9753, 130.4319)
  line L361 (177.5056, 130.9622) -> (188.1122, 120.3556) projected
  line L362 (188.1122, 120.3556) -> (186.3444, 118.5878) projected
  line L363 (186.8747, 176.2681) -> (187.5819, 176.9753)
  line L364 (188.1122, 177.5056) -> (186.3444, 175.7378) projected
  line L365 (186.8747, 119.1181) -> (187.5819, 119.8253)
  point P0 (0, 0)
  point P1 (153.35, 96.2)
  point P2 (267.65, 96.2)
  point P3 (381.95, 96.2)
  point P4 (496.25, 96.2)
  point P5 (369.25, 553.4)
  dimension "d33" = 3.175
  dimension "d34" = 457.2
  dimension "d35" = 25.4
  dimension "d36" = 457.2
  dimension "d37" = 57.15
  dimension "d40" = 114.3
  dimension "d45" = 3.175
  dimension "d46" = 457.2
  dimension "d49" = 0.5
  dimension "d50" = 0.5
  dimension "d51" = 0.5
  dimension "d52" = 0.5
  dimension "d55" = 114.3
  dimension "d58" = 57.15
  dimension "d61" = 0.5
  dimension "d62" = 0.5
  dimension "d63" = 0.5
  dimension "d64" = 0.5
  dimension "d67" = 114.3
  dimension "d70" = 57.15
  constraints: 656 end point, 28 collinear, 18 point on line, 15 parallel, 9 perpendicular, 6 horizontal, 5 midpoint, 2 vertical, 794 other
  measures "d33" distance of L2.end L3.end
  measures "d34" distance of L1.end L2.end
  measures "d35" distance of L7.end L8.end
  measures "d36" distance of L6.end L7.end
  measures "d37" distance of L3.end point (153.35, 96.2)
  measures "d40" distance of L6.end L10.start
  measures "d45" distance of L36.end L35.end
  measures "d46" distance of L35.end L34.end
  measures "d49" distance between parallel lines of L39 L42
  measures "d50" distance between parallel lines of L39 L43
  measures "d51" distance between parallel lines of L41 L44
  measures "d52" distance between parallel lines of L41 L45
  measures "d55" distance of L42.start L48.start
  measures "d58" distance of L42.start L60.start
  measures "d61" distance between parallel lines of L173 L176
  measures "d62" distance between parallel lines of L173 L177
  measures "d63" distance between parallel lines of L175 L178
  measures "d64" distance between parallel lines of L175 L179
  measures "d67" distance of L176.start L180.start
  measures "d70" distance of L176.start L192.start
extrude "Extrusion2" cut sketch "Sketch2" against normal blind 1
sketch "Sketch3" plane through (0, 2, 0) normal (0, 1, 0) x (1, 0, 0)
  line L0 (188.1122, 120.3556) -> (186.3444, 118.5878) construction
  line L1 (187.2283, 119.4717) -> (210.5, 96.2) construction
  line L2 (166.05, 96.2) -> (210.5, 96.2) construction
  line L3 (187.5819, 119.8253) -> (210.5, 96.9071)
  line L4 (186.8747, 119.1181) -> (209.7929, 96.2)
  line L5 (209.7929, 96.2) -> (210.5, 96.2)
  line L6 (210.5, 96.2) -> (210.5, 152.6429) projected
  line L7 (210.5, 96.9071) -> (210.5, 96.2)
  line L8 (186.8747, 119.1181) -> (187.5819, 119.8253)
  point P0 (0, 0)
  dimension "d76" = 0.5
  dimension "d77" = 0.5
  constraints: 14 end point, 3 collinear, 3 point on line, 2 parallel, 1 midpoint, 1 perpendicular
  measures "d76" distance between parallel lines of L1 L3
  measures "d77" distance between parallel lines of L1 L4
extrude "Extrusion3" cut sketch "Sketch3" against normal blind 1
pattern_linear "Rectangular Pattern2" count 4 spacing 114.3 along (1, 0, 0) of "Extrusion2"
ref_plane "Work Plane1" through (96.2, 0, -324.8) normal (0, 0, 1) x (1, 0, 0)
ref_plane "Work Plane2" through (324.8, 0, -96.2) normal (1, 0, 0) x (0, 0, -1)
split body "Split3" result two bodies by plane through (324.8, 0, -96.2) normal (1, 0, 0) first body at (332.2626, 0.5, -297.6981)
split body "Split4" result two bodies by plane through (96.2, 0, -324.8) normal (0, 0, 1) bodies 2 first body at (450.0981, 0.5, -103.6626)
split body "Split5" result two bodies by plane through (96.2, 0, -324.8) normal (0, 0, 1) bodies 3 first body at (221.4981, 0.5, -103.6626)
body "Solid4"
body "Solid5"
body "Solid6"
body "Solid7"
